Otrio_v5 (Autodesk Fusion 360 design; units mm, degrees)
Autodesk Fusion 360 part; units mm, degrees
ref_plane "WorkPlane1" through (0, 0, 4) normal (0, 0, 1) x (1, 0, 0)
sketch "Main Sketch1" plane through (0, 0, 4) normal (0, 0, 1) x (1, 0, 0)
  circle A0 centre (0, 0) radius 3
  circle A1 centre (0, 0) radius 5
  circle A2 centre (0, 0) radius 11
  circle A3 centre (0, 0) radius 13
  circle A4 centre (0, 0) radius 19
  circle A5 centre (-48, -96) radius 5
  circle A6 centre (-48, -96) radius 19
  circle A7 centre (-48, -96) radius 3
  circle A8 centre (-48, -96) radius 13
  circle A9 centre (-48, -96) radius 11
  circle A10 centre (0, -96) radius 5
  circle A11 centre (0, -96) radius 19
  circle A12 centre (0, -96) radius 3
  circle A13 centre (0, -96) radius 13
  circle A14 centre (0, -96) radius 11
  circle A15 centre (48, -96) radius 5
  circle A16 centre (48, -96) radius 19
  circle A17 centre (48, -96) radius 3
  circle A18 centre (48, -96) radius 13
  circle A19 centre (48, -96) radius 11
  circle A20 centre (-96, -48) radius 5
  circle A21 centre (-96, -48) radius 19
  circle A22 centre (-96, -48) radius 3
  circle A23 centre (-96, -48) radius 13
  circle A24 centre (-96, -48) radius 11
  circle A25 centre (-48, -48) radius 5
  circle A26 centre (-48, -48) radius 19
  circle A27 centre (-48, -48) radius 3
  circle A28 centre (-48, -48) radius 13
  circle A29 centre (-48, -48) radius 11
  circle A30 centre (0, -48) radius 5
  circle A31 centre (0, -48) radius 19
  circle A32 centre (0, -48) radius 3
  circle A33 centre (0, -48) radius 13
  circle A34 centre (0, -48) radius 11
  circle A35 centre (48, -48) radius 5
  circle A36 centre (48, -48) radius 19
  circle A37 centre (48, -48) radius 3
  circle A38 centre (48, -48) radius 13
  circle A39 centre (48, -48) radius 11
  circle A40 centre (96, -48) radius 5
  circle A41 centre (96, -48) radius 19
  circle A42 centre (96, -48) radius 3
  circle A43 centre (96, -48) radius 13
  circle A44 centre (96, -48) radius 11
  circle A45 centre (-96, 0) radius 5
  circle A46 centre (-96, 0) radius 19
  circle A47 centre (-96, 0) radius 3
  circle A48 centre (-96, 0) radius 13
  circle A49 centre (-96, 0) radius 11
  circle A50 centre (-48, 0) radius 5
  circle A51 centre (-48, 0) radius 19
  circle A52 centre (-48, 0) radius 3
  circle A53 centre (-48, 0) radius 13
  circle A54 centre (-48, 0) radius 11
  circle A55 centre (48, 0) radius 5
  circle A56 centre (48, 0) radius 19
  circle A57 centre (48, 0) radius 3
  circle A58 centre (48, 0) radius 13
  circle A59 centre (48, 0) radius 11
  circle A60 centre (96, 0) radius 5
  circle A61 centre (96, 0) radius 19
  circle A62 centre (96, 0) radius 3
  circle A63 centre (96, 0) radius 13
  circle A64 centre (96, 0) radius 11
  circle A65 centre (-96, 48) radius 5
  circle A66 centre (-96, 48) radius 19
  circle A67 centre (-96, 48) radius 3
  circle A68 centre (-96, 48) radius 13
  circle A69 centre (-96, 48) radius 11
  circle A70 centre (-48, 48) radius 5
  circle A71 centre (-48, 48) radius 19
  circle A72 centre (-48, 48) radius 3
  circle A73 centre (-48, 48) radius 13
  circle A74 centre (-48, 48) radius 11
  circle A75 centre (0, 48) radius 5
  circle A76 centre (0, 48) radius 19
  circle A77 centre (0, 48) radius 3
  circle A78 centre (0, 48) radius 13
  circle A79 centre (0, 48) radius 11
  circle A80 centre (48, 48) radius 5
  circle A81 centre (48, 48) radius 19
  circle A82 centre (48, 48) radius 3
  circle A83 centre (48, 48) radius 13
  circle A84 centre (48, 48) radius 11
  circle A85 centre (96, 48) radius 5
  circle A86 centre (96, 48) radius 19
  circle A87 centre (96, 48) radius 3
  circle A88 centre (96, 48) radius 13
  circle A89 centre (96, 48) radius 11
  circle A90 centre (-48, 96) radius 5
  circle A91 centre (-48, 96) radius 19
  circle A92 centre (-48, 96) radius 3
  circle A93 centre (-48, 96) radius 13
  circle A94 centre (-48, 96) radius 11
  circle A95 centre (0, 96) radius 5
  circle A96 centre (0, 96) radius 19
  circle A97 centre (0, 96) radius 3
  circle A98 centre (0, 96) radius 13
  circle A99 centre (0, 96) radius 11
  circle A100 centre (48, 96) radius 5
  circle A101 centre (48, 96) radius 19
  circle A102 centre (48, 96) radius 3
  circle A103 centre (48, 96) radius 13
  circle A104 centre (48, 96) radius 11
  line L0 (73, 73) -> (-73, 73)
  line L1 (-73, 73) -> (-73, -73)
  line L2 (-73, -73) -> (73, -73)
  line L3 (73, -73) -> (73, 73)
  line L4 (73, 73) -> (-73, -73) construction
  line L5 (-73, 73) -> (73, -73) construction
  line L6 (125, 125) -> (-125, -125) construction
  line L7 (-125, 125) -> (125, -125) construction
  dimension "d1" = 6
  dimension "d2" = 10
  dimension "d3" = 22
  dimension "d4" = 26
  dimension "d5" = 38
  dimension "d8" = 48
  dimension "d9" = 48
  dimension "d10" = 250
  dimension "d11" = 250
  constraint concentric A0 A1
  constraint concentric A1 A2
  constraint concentric A1 A3
  constraint concentric A3 A4
  constraint horizontal L0
  constraint perpendicular L0 L1
  constraint parallel L0 L2
  constraint parallel L1 L3
  constraint coincident L4 A0.centre
  constraint coincident L5 A0.centre
  constraint coincident A0.centre A1.centre
  constraint coincident L6 A0.centre
  constraint coincident L7 A0.centre
  measures "d1" diameter of A0
  measures "d2" diameter of A1
  measures "d3" diameter of A2
  measures "d4" diameter of A3
  measures "d5" diameter of A4
  measures "d10" distance of L6.end L7.end
  measures "d11" distance of L7.start L6.end
sketch "base" plane through (0, 0, 0) normal (0, 0, 1) x (1, 0, 0)
  line L0 (-125, 75) -> (-125, -75)
  line L1 (-75, -125) -> (75, -125)
  line L2 (125, -75) -> (125, 75)
  line L3 (125, 125) -> (-125, -125) construction
  line L4 (-125, 125) -> (125, -125) construction
  arc A0 (75, 125) -> (125, 75) centre (125, 125) ccw
  arc A1 (-125, 75) -> (-75, 125) centre (-125, 125) ccw
  arc A2 (-75, -125) -> (-125, -75) centre (-125, -125) ccw
  arc A3 (125, -75) -> (75, -125) centre (125, -125) ccw
  line L5 (-75, 125) -> (75, 125)
  dimension "d28" = 250
  dimension "d29" = 250
  dimension "d30" = 100
  dimension "d31" = 100
  dimension "d32" = 100
  dimension "d33" = 100
  constraint parallel L0 L2
  constraint coincident L3 origin
  constraint coincident L4 origin
  constraint coincident L3.end A2.centre
  constraint coincident L4.start A1.centre
  constraint coincident L3.start A0.centre
  constraint coincident L4.end A3.centre
  constraint horizontal L5
  measures "d28" distance of L3.end L4.end
  measures "d29" distance of L4.start L3.end
  measures "d30" diameter of A2
  measures "d31" diameter of A1
  measures "d32" diameter of A0
  measures "d33" diameter of A3
extrude "extrude main body" add sketch "base" along normal blind 6
extrude "cut groves" cut sketch "Main Sketch1" along normal blind 2 contours A0 | A2 | A4 | A6 | A7 | A9 | A11 | A12 | A14 | A16 | A17 | A19 | A21 | A22 | A24 | A26 | A27 | A29 | A31 | A32 | A34 | A36 | A37 | A39 | A41 | A42 | A44 | A46 | A47 | A49 | A51 | A52 | A54 | A56 | A57 | A59 | A61 | A62 | A64 | A66 | A67 | A69 | A71 | A72 | A74 | A76 | A77 | A79 | A81 | A82 | A84 | A86 | A87 | A89 | A91 | A92 | A94 | A96 | A97 | A99 | A101 | A102 | A104
sketch "text" plane through (0, 0, 0) normal (0, 0, 1) x (1, 0, 0)
  line L0 (-81.1, -79.3) -> (-81.1, -91.3) construction
  line L1 (-81.1, -91.3) -> (-74.1, -91.3) construction
  line L2 (-74.1, -91.3) -> (-74.1, -79.3) construction
  line L3 (-74.1, -79.3) -> (-81.1, -79.3) construction
  dimension "d43" = 8
equation "height = 6 mm"
equation "grooveheight = 2 mm"
equation "d27 = height - grooveheight"
equation "d34 = height"
equation "d36 = grooveheight"
named bodies: "main"
